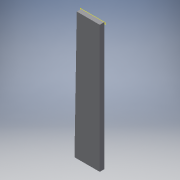
# Autodesk Inventor part: internalSupportBottom4
Saved by Autodesk Inventor 2019 (Build 230136000, 136)
## iProperties
Created: 2019-01-08
Part Number: internalSupportBottom4
Material: Wood (Birch)
Document SubType Name: Modeling
Designer: gaincarlo
Density: 0.55 g/cm^3
Appearance: Birch - Natural Polished
Author: gaincarlo
Autodesk Inventor part; units mm, degrees
ref_plane "YZ Plane" through (0, 0, 0) normal (1, 0, 0) x (0, 1, 0)
ref_plane "XZ Plane" through (0, 0, 0) normal (0, 1, 0) x (-1, 0, 0)
ref_plane "Work Plane1" through (0, 0, 0) normal (0, 0, 1) x (1, 0, 0)
sketch "Sketch1" plane through (0, 0, 0) normal (0, 0, 1) x (1, 0, 0)
  line L0 (-50, 3) -> (0, 3) construction
  line L1 (-57.9469, -274) -> (-52.9995, 3.0536) construction
  line L2 (-52.9995, 3.0536) -> (-50, 3) construction
  line L3 (-50, 3) -> (-54.9474, -274.0536) construction
  line L4 (-54.9474, -274.0536) -> (-57.9469, -274) construction
  line L5 (0, 3) -> (-50, 3)
  line L6 (-54.9474, -274.0536) -> (0, -274.0536)
  line L7 (0, -274.0536) -> (0, 3)
  line L8 (-54.9474, -274.0536) -> (-50, 3)
  point P0 (0, 0)
  constraints: 16 end point, 2 perpendicular, 1 collinear, 1 horizontal, 7 other
extrude "Extrusion1" add sketch "Sketch1" along normal blind 10
body "Solid1"
